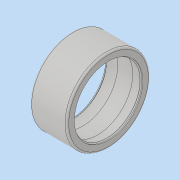
# Autodesk Inventor part: 橡胶外轮设计
Saved by Autodesk Inventor 2019 (Build 230136000, 136)
## iProperties
Created: 2020-10-29
Part Number: 橡胶外轮设计
Material: 常规
Document SubType Name: Modeling
Designer: Wang Hua
Density: 1 g/cm^3
Appearance: 默认
Author: Wang Hua
Autodesk Inventor part; units mm, degrees
ref_plane "YZ Plane" through (0, 0, 0) normal (1, 0, 0) x (0, 1, 0)
ref_plane "XZ Plane" through (0, 0, 0) normal (0, 1, 0) x (-1, 0, 0)
ref_plane "XY Plane" through (0, 0, 0) normal (0, 0, 1) x (1, 0, 0)
sketch "草图1" plane through (0, 0, 0) normal (0, 0, 1) x (1, 0, 0)
  line L0 (-10, 22.5) -> (10, 22.5)
  line L1 (-14, 0) -> (14, 0) projected
  line L2 (0, -4.5) -> (0, 27) projected
  line L3 (-10, 22.5) -> (-10, 18.5)
  line L4 (-10, 18.5) -> (-9.5, 18.5)
  arc A0 (-9, 18) -> (-9.5, 18.5) centre (-9.5, 18) ccw
  line L5 (-9.5, 18) -> (-7.8897, 18) construction
  arc A1 (-4.0742, 19) -> (-9, 18) centre (-4.4094, 8.0196) ccw
  line L6 (10, 22.5) -> (10, 18.5)
  line L7 (10, 18.5) -> (9.5, 18.5)
  arc A2 (9.5, 18.5) -> (9, 18) centre (9.5, 18) ccw
  arc A3 (9, 18) -> (4.0742, 19) centre (4.4094, 8.0196) ccw
  line L8 (-4.0742, 19) -> (4.0742, 19)
  point P0 (0, 0)
  dimension "d0" = 20
  dimension "d1" = 0.5
  dimension "d2" = 4
  dimension "d3" = 1
  dimension "d4" = 22.5
  dimension "d5" = 18
  dimension "d6" = 19
  dimension "d7" = 10.9856
  dimension "d8" = 8.1484
  constraints: 14 end point, 8 point on circle, 7 symmetric about line, 4 centre point, 3 horizontal, 1 parallel, 1 point on line, 1 vertical, 2 other
  measures "d0" distance of L0.start L0.end
  measures "d1" distance of L3.end L4.end
  measures "d2" distance of L0.start L3.end
  measures "d3" diameter of A0
  measures "d4" distance between parallel lines of L1 L0
  measures "d5" distance from line of L1 A2.end
  measures "d6" distance between parallel lines of L1 L8
  measures "d7" radius of A1
  measures "d8" distance of L8.start L8.end
revolve "旋转1" add sketch "草图1" angle 360 about axis through (-10, 0, 0) along (1, 0, 0)
fillet "圆角1" radius 1 2 edges at (-10, -22.5, 0) (10, -22.5, 0)
